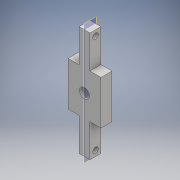
# Autodesk Inventor part: Support poulie
Saved by Autodesk Inventor 2018 (Build 220112000, 112)
## iProperties
Created: 2018-05-14
Part Number: Support poulie
Material: Générique
Document SubType Name: Modeling
Designer: Dimitri
Density: 1 g/cm^3
Appearance: Par défaut
Author: Dimitri
Autodesk Inventor part; units mm, degrees
ref_plane "YZ Plane" through (0, 0, 0) normal (1, 0, 0) x (0, 1, 0)
ref_plane "XZ Plane" through (0, 0, 0) normal (0, 1, 0) x (-1, 0, 0)
ref_plane "XY Plane" through (0, 0, 0) normal (0, 0, 1) x (1, 0, 0)
sketch "Esquisse1" plane through (0, 0, 0) normal (0, 1, 0) x (-1, 0, 0)
  line L0 (-5, 50) -> (5, 50)
  line L1 (5, 50) -> (5, -50)
  line L2 (5, -50) -> (-5, -50)
  line L3 (-5, -50) -> (-5, 50)
  line L4 (-5, 50) -> (5, -50) construction
  line L5 (5, 50) -> (-5, -50) construction
  point P0 (0, 0)
  dimension "d0" = 10
  dimension "d1" = 100
  constraints: 12 end point, 2 midpoint, 2 parallel, 1 horizontal, 1 perpendicular
  measures "d0" distance of L1.end L2.end
  measures "d1" distance of L0.end L1.end
extrude "Extrusion1" add sketch "Esquisse1" along normal blind 10
sketch "Esquisse2" plane through (-5, 0, -50) normal (-1, 0, 0) x (0, 0, 1)
  line L0 (0, 0) -> (100, 0) projected
  line L1 (100, 0) -> (100, 10) projected
  point P0 (50, 0)
  point P1 (5, 5)
  point P2 (95, 5)
hole "Perçage1" at (-5, 5, -45) at (-5, 5, 45) direction (1, 0, 0) diameter 5 end through all
sketch "Esquisse4" plane through (-5, 0, -50) normal (-1, 0, 0) x (0, 0, 1)
  line L0 (100, 10) -> (0, 10) projected
  line L1 (30, 10) -> (70, 10)
  line L2 (70, 10) -> (70, 0)
  line L3 (0, 0) -> (100, 0) projected
  line L4 (70, 0) -> (30, 0)
  line L5 (30, 0) -> (30, 10)
  point P0 (50, 0)
  constraints: 8 end point, 3 point on line, 1 parallel
extrude "Extrusion2" add sketch "Esquisse4" along normal blind 10
mirror "Symétrie1" about plane through (0, 0, 0) normal (1, 0, 0) of "Extrusion2"
sketch "Esquisse5" plane through (0, 10, 0) normal (0, 1, 0) x (1, 0, 0)
  point P0 (0, 0)
  point P1 (0, 0)
  constraints: 1 coincident
hole "Perçage2" at (0, 10, 0) direction (0, -1, 0) diameter 9 end through all
ref_plane "Plan de construction1" through (0, 0, 0) normal (1, 0, 0) x (0, 1, 0)
